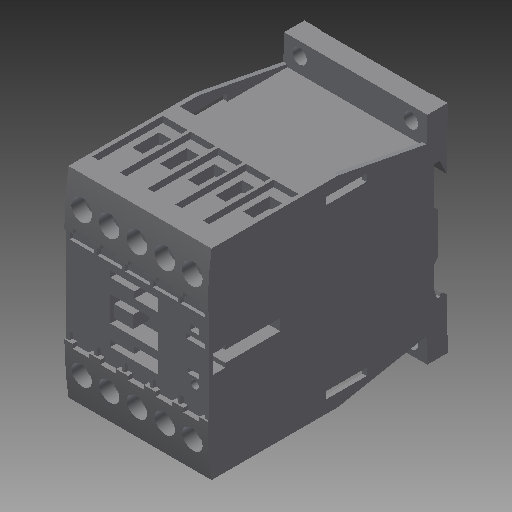
# Autodesk Inventor part: 276845
Saved by Autodesk Inventor 2019.3 (Build 233278000, 278)
## iProperties
Category: PARTsolutions
Company: MOELLER
Created: 2018-10-25
Part Number: 276845
Material: Generic
Catalog Web Link: www.cadenas.de
Description: DC operated-
Vendor: MOELLER
Document SubType Name: Modeling
Designer: psadmin
Manufacturer: MOELLER
Mass: 179.978 g
Surface Area: 287.285 cm^2
Volume: 179.978 cm^3
Density: 1 g/cm^3
Appearance: PSOLRGB-175-175-175
PSOL_IDENT_0: {$CADENAS_DATA\23d-libs\moeller\2\695\733\735\737\740.prj},171 {VTYP=3D},{NB=276845},{LINA=276845},{
PSOL_IDENT_1: NN=DC operated},{DATE=04.10.2018 12:16:44},{GEOMDATE=04.10.2018 08:29:25},{VERSION=v181004082925},{L
PSOL_IDENT_2: INEID=650},{WBVAR=},{WBNUMERIC=}  {NB=276845},{LINA=276845},{KT=DUMMY},{PFOTO=2110pic-214.jpg},{PLID=
PSOL_IDENT_3: 276845},{DATA_SHEET=Data sheet},{MANUTYPEDESC=DILM12-10(24VDC)},{DESCSHORT=Contactor, 3p+1N/O, 5.5kW
PSOL_IDENT_4: /400V/AC3},{DESCLONG=Contactor, Application: Contactors for Motors, Contactors up to 170 A, 3 pole,
PSOL_IDENT_5: Utilization category: AC-1: Non-inductive or slightly inductive loads, resistance furnaces, NAC-3: N
PSOL_IDENT_6: ormal AC induction motors: starting, switch off during running, AC-4: Normal AC induction motors: st
PSOL_IDENT_7: arting, plugging, reversing, inching, Connection technique: Screw terminals, Notes: Also suitable fo
PSOL_IDENT_8: r motors with efficiency class IE3., IE3-ready devices are identified by the logo on their packaging
PSOL_IDENT_9: ., Number of poles: 3 pole, Rated operational current AC-3 380 V 400 V: Ie= 12 A, Rated operational
PSOL_IDENT_10: current AC-1 Conventional free air thermal current, 3 pole, 50 - 60 Hz Open at 40 °C: Ith =Ie= 22 A,
PSOL_IDENT_11: enclosed: Ith= 18 A, Rated operational current AC-1 Conventional free air thermal current, 1 pole o
PSOL_IDENT_12: pen: Ith= 50 A, enclosed: Ith= 45 A, Max. rating for three-phase motors, 50 - 60 Hz AC-3 220 V 230 V
PSOL_IDENT_13: : P= 3.5 kW, 380 V 400 V: P= 5.5 kW, 660 V 690 V: P= 6.5 kW, Max. rating for three-phase motors, 50
PSOL_IDENT_14: - 60 Hz AC-4 220 V 230 V: P= 2 kW, 380 V 400 V: P= 3 kW, 660 V 690 V: P= 4.4 kW, Can be combined wit
PSOL_IDENT_15: h auxiliary contact: DILM32-XHI.., DILA-XHI(V).., Contacts N/O = Normally open: 1 N/O, Instructions:
PSOL_IDENT_16: Contacts to EN 50 012., Integrated varistor suppressor circuit., Voltage AC/DC: DC operation},{EAN=
PSOL_IDENT_17: 4015082768454},{ECLASS_8_1=27-37-10-03},{PACKAGED_WEIGHT=0.296},{DATA_SHEET_=http://datasheet.moelle
PSOL_IDENT_18: r.net/datasheet.php?model=276845&locale=en_GB},{DATA_SHEET_ENG=http://datasheet.moeller.net/datashee
PSOL_IDENT_19: t.php?model=276845&locale=en_GB},{DATA_SHEET_DEU=http://datasheet.moeller.net/datasheet.php?model=27
PSOL_IDENT_20: 6845&locale=de_DE}
NN: DC operated
NB: 276845
NBSYN: $PLID.
LINA: 276845
PFOTO: 2110pic-214.jpg
PLID: 276845
DATA_SHEET: Data sheet
MANUTYPEDESC: DILM12-10(24VDC)
DESCSHORT: Contactor, 3p+1N/O, 5.5kW/400V/AC3
DESCLONG: Contactor, Application: Contactors for Motors, Contactors up to 170 A, 3 pole, Utilization category: AC-1: Non-inductive or slightly inductive loads, resistance furnaces, NAC-3: Normal AC induction motors: starting, switch off during running, AC-4: Normal AC induction motors: starting, plugging, reversing, inching, Connection technique: Screw terminals, Notes: Also suitable for motors with efficiency class IE3., IE3-ready devices are identified by the logo on their packaging., Number of poles: 3 pole, Rated operational current AC-3 380 V 400 V: Ie= 12 A, Rated operational current AC-1 Conventional free air thermal current, 3 pole, 50 - 60 Hz Open at 40 °C: Ith =Ie= 22 A, enclosed: Ith= 18 A, Rated operational current AC-1 Conventional free air thermal current, 1 pole open: Ith= 50 A, enclosed: Ith= 45 A, Max. rating for three-phase motors, 50 - 60 Hz AC-3 220 V 230 V: P= 3.5 kW, 380 V 400 V: P= 5.5 kW, 660 V 690 V: P= 6.5 kW, Max. rating for three-phase motors, 50 - 60 Hz AC-4 220 V 230 V: P= 2 kW, 380 V 400 V: P= 3 kW, 660 V 690 V: P= 4.4 kW, Can be combined with auxiliary contact: DILM32-XHI.., DILA-XHI(V).., Contacts N/O = Normally open: 1 N/O, Instructions: Contacts to EN 50 012., Integrated varistor suppressor circuit., Voltage AC/DC: DC operation
EAN: 4015082768454
ECLASS_8_1: 27-37-10-03
PACKAGED_WEIGHT: 0.296
SUPPLIER: MOELLER
ARTICLENO: 276845
BOMINFO: 276845
CREATOR: CADENAS GmbH
Title: 276845
Author: Cadenas PARTsolutions
Autodesk Inventor part; units mm, degrees
sketch "Sketch_1" plane through (0, 0, 0) normal (1, 0, 0) x (0, 1, 0)
  arc A0 (-15, 72.4777) -> (-31.5, 71.2047) centre (-12.5, -67.5) ccw
  line L0 (-31.5, 71.2047) -> (-31.5, 31.404)
  line L1 (-31.5, 31.404) -> (-26.1094, 3.6715)
  line L2 (-26.1094, 3.6715) -> (-34, 3.396)
  line L3 (-34, 3.396) -> (-34, -3)
  line L4 (-34, -3) -> (-17.9929, -3)
  line L5 (-17.9929, -3) -> (-16.5, -0.8679)
  line L6 (-16.5, -0.8679) -> (-17.5, -0.6)
  line L7 (-17.5, -0.6) -> (-17.5, 0.3)
  line L8 (-17.5, 0.3) -> (-15.0273, 1.2)
  line L9 (-15.0273, 1.2) -> (-7.7, 1.2)
  line L10 (-7.7, 1.2) -> (-6.5, 0)
  line L11 (-6.5, 0) -> (6.5, 0)
  line L12 (6.5, 0) -> (7.7, 1.2)
  line L13 (7.7, 1.2) -> (19.5, 1.2)
  line L14 (19.5, 1.2) -> (19.5, -0.5)
  line L15 (19.5, -0.5) -> (15, -2.5984)
  line L16 (15, -2.5984) -> (15, -3)
  line L17 (15, -3) -> (34, -3)
  line L18 (34, -3) -> (34, 3.396)
  line L19 (34, 3.396) -> (26.1094, 3.6715)
  line L20 (26.1094, 3.6715) -> (31.5, 31.404)
  line L21 (31.5, 31.404) -> (31.5, 71.2047)
  arc A1 (31.5, 71.2047) -> (15, 72.4777) centre (12.5, -67.5) ccw
  line L22 (15, 72.4777) -> (15, 72)
  line L23 (15, 72) -> (-15, 72)
  line L24 (-15, 72) -> (-15, 72.4777)
  line L25 (27.55, 35.25) -> (25.3, 35.25)
  line L26 (25.3, 35.25) -> (25.3, 22.5)
  line L27 (25.3, 22.5) -> (27.55, 22.5)
  line L28 (27.55, 22.5) -> (27.55, 35.25)
  line L29 (-27.55, 35.25) -> (-27.55, 22.5)
  line L30 (-27.55, 22.5) -> (-25.3, 22.5)
  line L31 (-25.3, 22.5) -> (-25.3, 35.25)
  line L32 (-25.3, 35.25) -> (-27.55, 35.25)
  constraints: 66 end point, 4 point on circle, 2 centre point
extrude "Extrusion1" add sketch "Sketch_1" along normal blind 45
sketch "Sketch_77" plane through (0, 0, -3) normal (0, 0, 1) x (1, 0, 0)
  line L0 (0, 29) -> (0, -29)
  line L1 (0, -29) -> (1.3, -29)
  line L2 (1.3, -29) -> (1.3, -32.7)
  line L3 (1.3, -32.7) -> (5, -32.7)
  line L4 (5, -32.7) -> (5, -34)
  line L5 (5, -34) -> (40, -34)
  line L6 (40, -34) -> (40, -32.7)
  line L7 (40, -32.7) -> (43.7, -32.7)
  line L8 (43.7, -32.7) -> (43.7, -29)
  line L9 (43.7, -29) -> (45, -29)
  line L10 (45, -29) -> (45, 29)
  line L11 (45, 29) -> (43.7, 29)
  line L12 (43.7, 29) -> (43.7, 32.7)
  line L13 (43.7, 32.7) -> (40, 32.7)
  line L14 (40, 32.7) -> (40, 34)
  line L15 (40, 34) -> (5, 34)
  line L16 (5, 34) -> (5, 32.7)
  line L17 (5, 32.7) -> (1.3, 32.7)
  line L18 (1.3, 32.7) -> (1.3, 29)
  line L19 (1.3, 29) -> (0, 29)
  constraints: 40 end point
extrude "Extrusion2" cut sketch "Sketch_77" along normal mid plane 0.4
sketch "Sketch_2" plane through (0, 0, -5) normal (0, 0, 1) x (1, 0, 0)
  line L0 (15, -44) -> (30, -44)
  line L1 (30, -44) -> (30, -10)
  line L2 (30, -10) -> (15, -10)
  line L3 (15, -10) -> (15, -44)
  constraints: 8 end point
extrude "Extrusion3" cut sketch "Sketch_2" along normal blind 6.2
sketch "Sketch_3" plane through (0, 0, 0) normal (0, 0, 1) x (1, 0, 0)
  line L0 (14.8, -59.3) -> (30.2, -59.3)
  line L1 (30.2, -59.3) -> (30.2, -25.3)
  line L2 (30.2, -25.3) -> (14.8, -25.3)
  line L3 (14.8, -25.3) -> (14.8, -59.3)
  constraints: 8 end point
extrude "Extrusion4" cut sketch "Sketch_3" along normal mid plane 10
sketch "Sketch_4" plane through (22.5, 0, 0) normal (1, 0, 0) x (0, 0, -1)
  line L0 (-37.5, 25.3) -> (-3.6998, 25.3)
  line L1 (-3.6998, 25.3) -> (-3.396, 34)
  line L2 (-3.396, 34) -> (-37.5, 34)
  line L3 (-37.5, 34) -> (-37.5, 25.3)
  constraints: 8 end point
extrude "Extrusion5" cut sketch "Sketch_4" along normal mid plane 42.4
sketch "Sketch_5" plane through (22.5, 0, 0) normal (1, 0, 0) x (0, 0, -1)
  line L0 (-37.5, -25.3) -> (-37.5, -34)
  line L1 (-37.5, -34) -> (-3.396, -34)
  line L2 (-3.396, -34) -> (-3.6998, -25.3)
  line L3 (-3.6998, -25.3) -> (-37.5, -25.3)
  constraints: 8 end point
extrude "Extrusion6" cut sketch "Sketch_5" along normal mid plane 42.4
sketch "Sketch_6" plane through (0, 0, 0) normal (0, 0, 1) x (1, 0, 0)
  circle A0 centre (22.5, 0) radius 4
  constraints: 1 centre point
extrude "Extrusion7" add sketch "Sketch_6" against normal blind 1
sketch "Sketch_7" plane through (0, 31.5, 0) normal (0, 1, 0) x (1, 0, 0)
  line L0 (1.2, -42.7) -> (1.2, -64.9)
  line L1 (1.2, -64.9) -> (9, -64.9)
  line L2 (9, -64.9) -> (9, -42.7)
  line L3 (9, -42.7) -> (1.2, -42.7)
  constraints: 8 end point
extrude "Extrusion8" cut sketch "Sketch_7" against normal blind 2
sketch "Sketch_8" plane through (0, 31.5, 0) normal (0, 1, 0) x (1, 0, 0)
  line L0 (9.9, -42.7) -> (9.9, -64.9)
  line L1 (9.9, -64.9) -> (17.7, -64.9)
  line L2 (17.7, -64.9) -> (17.7, -42.7)
  line L3 (17.7, -42.7) -> (9.9, -42.7)
  constraints: 8 end point
extrude "Extrusion9" cut sketch "Sketch_8" against normal blind 2
sketch "Sketch_9" plane through (0, 31.5, 0) normal (0, 1, 0) x (1, 0, 0)
  line L0 (18.6, -42.7) -> (18.6, -64.9)
  line L1 (18.6, -64.9) -> (26.4, -64.9)
  line L2 (26.4, -64.9) -> (26.4, -42.7)
  line L3 (26.4, -42.7) -> (18.6, -42.7)
  constraints: 8 end point
extrude "Extrusion10" cut sketch "Sketch_9" against normal blind 2
sketch "Sketch_10" plane through (0, 31.5, 0) normal (0, 1, 0) x (1, 0, 0)
  line L0 (27.3, -42.7) -> (27.3, -64.9)
  line L1 (27.3, -64.9) -> (35.1, -64.9)
  line L2 (35.1, -64.9) -> (35.1, -42.7)
  line L3 (35.1, -42.7) -> (27.3, -42.7)
  constraints: 8 end point
extrude "Extrusion11" cut sketch "Sketch_10" against normal blind 2
sketch "Sketch_11" plane through (0, 31.5, 0) normal (0, 1, 0) x (1, 0, 0)
  line L0 (36, -42.7) -> (36, -64.9)
  line L1 (36, -64.9) -> (43.8, -64.9)
  line L2 (43.8, -64.9) -> (43.8, -42.7)
  line L3 (43.8, -42.7) -> (36, -42.7)
  constraints: 8 end point
extrude "Extrusion12" cut sketch "Sketch_11" against normal blind 2
sketch "Sketch_12" plane through (0, -31.5, 0) normal (0, 1, 0) x (1, 0, 0)
  line L0 (1.2, -42.7) -> (1.2, -64.9)
  line L1 (1.2, -64.9) -> (9, -64.9)
  line L2 (9, -64.9) -> (9, -42.7)
  line L3 (9, -42.7) -> (1.2, -42.7)
  constraints: 8 end point
sketch "Sketch_13" plane through (0, -31.5, 0) normal (0, 1, 0) x (1, 0, 0)
  line L0 (9.9, -42.7) -> (9.9, -64.9)
  line L1 (9.9, -64.9) -> (17.7, -64.9)
  line L2 (17.7, -64.9) -> (17.7, -42.7)
  line L3 (17.7, -42.7) -> (9.9, -42.7)
  constraints: 8 end point
sketch "Sketch_14" plane through (0, -31.5, 0) normal (0, 1, 0) x (1, 0, 0)
  line L0 (18.6, -42.7) -> (18.6, -64.9)
  line L1 (18.6, -64.9) -> (26.4, -64.9)
  line L2 (26.4, -64.9) -> (26.4, -42.7)
  line L3 (26.4, -42.7) -> (18.6, -42.7)
  constraints: 8 end point
sketch "Sketch_15" plane through (0, -31.5, 0) normal (0, 1, 0) x (1, 0, 0)
  line L0 (27.3, -42.7) -> (27.3, -64.9)
  line L1 (27.3, -64.9) -> (35.1, -64.9)
  line L2 (35.1, -64.9) -> (35.1, -42.7)
  line L3 (35.1, -42.7) -> (27.3, -42.7)
  constraints: 8 end point
sketch "Sketch_16" plane through (0, -31.5, 0) normal (0, 1, 0) x (1, 0, 0)
  line L0 (36, -42.7) -> (36, -64.9)
  line L1 (36, -64.9) -> (43.8, -64.9)
  line L2 (43.8, -64.9) -> (43.8, -42.7)
  line L3 (43.8, -42.7) -> (36, -42.7)
  constraints: 8 end point
extrude "Extrusion13" cut sketch "Sketch_12" along normal blind 2
extrude "Extrusion14" cut sketch "Sketch_13" along normal blind 2
extrude "Extrusion15" cut sketch "Sketch_16" along normal blind 2
extrude "Extrusion16" cut sketch "Sketch_15" along normal blind 2
extrude "Extrusion17" cut sketch "Sketch_14" along normal blind 2
sketch "Sketch_17" plane through (0, 31.5, 0) normal (0, 1, 0) x (1, 0, 0)
  line L0 (3.1, -45.8) -> (3.1, -54.2)
  line L1 (3.1, -54.2) -> (7.1, -54.2)
  line L2 (7.1, -54.2) -> (7.1, -45.8)
  line L3 (7.1, -45.8) -> (3.1, -45.8)
  constraints: 8 end point
extrude "Extrusion18" cut sketch "Sketch_17" against normal blind 5.3
sketch "Sketch_18" plane through (0, 31.5, 0) normal (0, 1, 0) x (1, 0, 0)
  line L0 (11.8, -45.8) -> (11.8, -54.2)
  line L1 (11.8, -54.2) -> (15.8, -54.2)
  line L2 (15.8, -54.2) -> (15.8, -45.8)
  line L3 (15.8, -45.8) -> (11.8, -45.8)
  constraints: 8 end point
extrude "Extrusion19" cut sketch "Sketch_18" against normal blind 5.3
sketch "Sketch_19" plane through (0, 31.5, 0) normal (0, 1, 0) x (1, 0, 0)
  line L0 (20.5, -45.8) -> (20.5, -54.2)
  line L1 (20.5, -54.2) -> (24.5, -54.2)
  line L2 (24.5, -54.2) -> (24.5, -45.8)
  line L3 (24.5, -45.8) -> (20.5, -45.8)
  constraints: 8 end point
extrude "Extrusion20" cut sketch "Sketch_19" against normal blind 5.3
sketch "Sketch_20" plane through (0, 31.5, 0) normal (0, 1, 0) x (1, 0, 0)
  line L0 (29.2, -45.8) -> (29.2, -54.2)
  line L1 (29.2, -54.2) -> (33.2, -54.2)
  line L2 (33.2, -54.2) -> (33.2, -45.8)
  line L3 (33.2, -45.8) -> (29.2, -45.8)
  constraints: 8 end point
extrude "Extrusion21" cut sketch "Sketch_20" against normal blind 5.3
sketch "Sketch_21" plane through (0, 31.5, 0) normal (0, 1, 0) x (1, 0, 0)
  line L0 (37.9, -45.8) -> (37.9, -54.2)
  line L1 (37.9, -54.2) -> (41.9, -54.2)
  line L2 (41.9, -54.2) -> (41.9, -45.8)
  line L3 (41.9, -45.8) -> (37.9, -45.8)
  constraints: 8 end point
extrude "Extrusion22" cut sketch "Sketch_21" against normal blind 5.3
sketch "Sketch_22" plane through (0, -31.5, 0) normal (0, 1, 0) x (1, 0, 0)
  line L0 (3.1, -45.8) -> (3.1, -54.2)
  line L1 (3.1, -54.2) -> (7.1, -54.2)
  line L2 (7.1, -54.2) -> (7.1, -45.8)
  line L3 (7.1, -45.8) -> (3.1, -45.8)
  constraints: 8 end point
extrude "Extrusion23" cut sketch "Sketch_22" along normal blind 5.3
sketch "Sketch_23" plane through (0, -31.5, 0) normal (0, 1, 0) x (1, 0, 0)
  line L0 (37.9, -45.8) -> (37.9, -54.2)
  line L1 (37.9, -54.2) -> (41.9, -54.2)
  line L2 (41.9, -54.2) -> (41.9, -45.8)
  line L3 (41.9, -45.8) -> (37.9, -45.8)
  constraints: 8 end point
extrude "Extrusion24" cut sketch "Sketch_23" along normal blind 5.3
sketch "Sketch_24" plane through (0, -31.5, 0) normal (0, 1, 0) x (1, 0, 0)
  line L0 (29.2, -45.8) -> (29.2, -54.2)
  line L1 (29.2, -54.2) -> (33.2, -54.2)
  line L2 (33.2, -54.2) -> (33.2, -45.8)
  line L3 (33.2, -45.8) -> (29.2, -45.8)
  constraints: 8 end point
extrude "Extrusion25" cut sketch "Sketch_24" along normal blind 5.3
sketch "Sketch_25" plane through (0, -31.5, 0) normal (0, 1, 0) x (1, 0, 0)
  line L0 (20.5, -45.8) -> (20.5, -54.2)
  line L1 (20.5, -54.2) -> (24.5, -54.2)
  line L2 (24.5, -54.2) -> (24.5, -45.8)
  line L3 (24.5, -45.8) -> (20.5, -45.8)
  constraints: 8 end point
extrude "Extrusion26" cut sketch "Sketch_25" along normal blind 5.3
sketch "Sketch_26" plane through (0, -31.5, 0) normal (0, 1, 0) x (1, 0, 0)
  line L0 (11.8, -45.8) -> (11.8, -54.2)
  line L1 (11.8, -54.2) -> (15.8, -54.2)
  line L2 (15.8, -54.2) -> (15.8, -45.8)
  line L3 (15.8, -45.8) -> (11.8, -45.8)
  constraints: 8 end point
extrude "Extrusion27" cut sketch "Sketch_26" along normal blind 5.3
sketch "Sketch_27" plane through (0, 0, 66.95) normal (0, 0, 1) x (1, 0, 0)
  circle A0 centre (5.1, 22.5) radius 3.2
  constraints: 1 centre point
extrude "Extrusion28" cut sketch "Sketch_27" along normal blind 10
sketch "Sketch_52" plane through (0, 0, 66.95) normal (0, 0, 1) x (1, 0, 0)
  circle A0 centre (13.8, -22.5) radius 3.2
  constraints: 1 centre point
extrude "Extrusion29" cut sketch "Sketch_52" along normal blind 10
sketch "Sketch_28" plane through (0, 0, 66.95) normal (0, 0, 1) x (1, 0, 0)
  circle A0 centre (13.8, 22.5) radius 3.2
  constraints: 1 centre point
extrude "Extrusion30" cut sketch "Sketch_28" along normal blind 10
sketch "Sketch_46" plane through (0, 0, 66.95) normal (0, 0, 1) x (1, 0, 0)
  circle A0 centre (22.5, 22.5) radius 3.2
  constraints: 1 centre point
extrude "Extrusion31" cut sketch "Sketch_46" along normal blind 10
sketch "Sketch_47" plane through (0, 0, 66.95) normal (0, 0, 1) x (1, 0, 0)
  circle A0 centre (31.2, 22.5) radius 3.2
  constraints: 1 centre point
extrude "Extrusion32" cut sketch "Sketch_47" along normal blind 10
sketch "Sketch_48" plane through (0, 0, 66.95) normal (0, 0, 1) x (1, 0, 0)
  circle A0 centre (39.9, 22.5) radius 3.2
  constraints: 1 centre point
extrude "Extrusion33" cut sketch "Sketch_48" along normal blind 10
sketch "Sketch_49" plane through (0, 0, 66.95) normal (0, 0, 1) x (1, 0, 0)
  circle A0 centre (39.9, -22.5) radius 3.2
  constraints: 1 centre point
extrude "Extrusion34" cut sketch "Sketch_49" along normal blind 10
sketch "Sketch_50" plane through (0, 0, 66.95) normal (0, 0, 1) x (1, 0, 0)
  circle A0 centre (31.2, -22.5) radius 3.2
  constraints: 1 centre point
extrude "Extrusion35" cut sketch "Sketch_50" along normal blind 10
sketch "Sketch_51" plane through (0, 0, 66.95) normal (0, 0, 1) x (1, 0, 0)
  circle A0 centre (22.5, -22.5) radius 3.2
  constraints: 1 centre point
extrude "Extrusion36" cut sketch "Sketch_51" along normal blind 10
sketch "Sketch_53" plane through (0, 0, 66.95) normal (0, 0, 1) x (1, 0, 0)
  circle A0 centre (5.1, -22.5) radius 3.2
  constraints: 1 centre point
extrude "Extrusion37" cut sketch "Sketch_53" along normal blind 10
sketch "Sketch_29" plane through (0, 0, 66.95) normal (0, 0, 1) x (1, 0, 0)
  circle A0 centre (5.1, 22.5) radius 3.8
  line L0 (2.825, 23) -> (2.825, 22)
  line L1 (2.825, 22) -> (4.6, 22)
  line L2 (4.6, 22) -> (4.6, 19.2)
  line L3 (4.6, 19.2) -> (5.6, 19.2)
  line L4 (5.6, 19.2) -> (5.6, 22)
  line L5 (5.6, 22) -> (7.375, 22)
  line L6 (7.375, 22) -> (7.375, 23)
  line L7 (7.375, 23) -> (5.6, 23)
  line L8 (5.6, 23) -> (5.6, 25.8)
  line L9 (5.6, 25.8) -> (4.6, 25.8)
  line L10 (4.6, 25.8) -> (4.6, 23)
  line L11 (4.6, 23) -> (2.825, 23)
  constraints: 24 end point, 1 centre point
extrude "Extrusion38" add sketch "Sketch_29" along normal blind 1.1
sketch "Sketch_31" plane through (0, 0, 71) normal (0, 0, 1) x (1, 0, 0)
  line L0 (1.2, 15) -> (1.2, 12.5)
  line L1 (1.2, 12.5) -> (9, 12.5)
  line L2 (9, 12.5) -> (9, 15)
  line L3 (9, 15) -> (7.6, 15)
  line L4 (7.6, 15) -> (7.6, 16.3)
  line L5 (7.6, 16.3) -> (2.6, 16.3)
  line L6 (2.6, 16.3) -> (2.6, 15)
  line L7 (2.6, 15) -> (1.2, 15)
  constraints: 16 end point
extrude "Extrusion39" cut sketch "Sketch_31" along normal blind 6
sketch "Sketch_33" plane through (0, 0, 71) normal (0, 0, 1) x (1, 0, 0)
  line L0 (1.2, -15) -> (2.6, -15)
  line L1 (2.6, -15) -> (2.6, -16.3)
  line L2 (2.6, -16.3) -> (7.6, -16.3)
  line L3 (7.6, -16.3) -> (7.6, -15)
  line L4 (7.6, -15) -> (9, -15)
  line L5 (9, -15) -> (9, -12.5)
  line L6 (9, -12.5) -> (1.2, -12.5)
  line L7 (1.2, -12.5) -> (1.2, -15)
  constraints: 16 end point
extrude "Extrusion40" cut sketch "Sketch_33" along normal blind 6
sketch "Sketch_35" plane through (0, 0, 72) normal (0, 0, 1) x (1, 0, 0)
  line L0 (14, 4) -> (14, -4)
  line L1 (14, -4) -> (29, -4)
  line L2 (29, -4) -> (29, 4)
  line L3 (29, 4) -> (14, 4)
  line L4 (15.15, 1.95) -> (15.15, -1.95)
  line L5 (15.15, -1.95) -> (21.15, -1.95)
  line L6 (21.15, -1.95) -> (21.15, 1.95)
  line L7 (21.15, 1.95) -> (15.15, 1.95)
  constraints: 16 end point
extrude "Extrusion41" cut sketch "Sketch_35" against normal blind 5
sketch "Sketch_36" plane through (0, 0, 72) normal (0, 0, 1) x (1, 0, 0)
  line L0 (14, 8.5) -> (21.5, 8.5)
  line L1 (21.5, 8.5) -> (21.5, 6.5)
  line L2 (21.5, 6.5) -> (29, 6.5)
  line L3 (29, 6.5) -> (29, 10.4)
  line L4 (29, 10.4) -> (14, 10.4)
  line L5 (14, 10.4) -> (14, 8.5)
  constraints: 12 end point
extrude "Extrusion42" cut sketch "Sketch_36" against normal blind 5
sketch "Sketch_37" plane through (0, 0, 72) normal (0, 0, 1) x (1, 0, 0)
  line L0 (14, -8.5) -> (14, -10.4)
  line L1 (14, -10.4) -> (29, -10.4)
  line L2 (29, -10.4) -> (29, -6.5)
  line L3 (29, -6.5) -> (21.5, -6.5)
  line L4 (21.5, -6.5) -> (21.5, -8.5)
  line L5 (21.5, -8.5) -> (14, -8.5)
  constraints: 12 end point
extrude "Extrusion43" cut sketch "Sketch_37" against normal blind 5
sketch "Sketch_38" plane through (0, 0, 72) normal (0, 0, 1) x (1, 0, 0)
  line L0 (37.9, 5.3) -> (37.9, 3.9)
  line L1 (37.9, 3.9) -> (43.6, 3.9)
  line L2 (43.6, 3.9) -> (43.6, 5.3)
  line L3 (43.6, 5.3) -> (37.9, 5.3)
  constraints: 8 end point
extrude "Extrusion44" cut sketch "Sketch_38" against normal blind 4
sketch "Sketch_78" plane through (0, 0, 72) normal (0, 0, 1) x (1, 0, 0)
  line L0 (39, 8.4) -> (39, 6.7)
  line L1 (39, 6.7) -> (42, 6.7)
  line L2 (42, 6.7) -> (42, 8.4)
  line L3 (42, 8.4) -> (39, 8.4)
  constraints: 8 end point
extrude "Extrusion45" cut sketch "Sketch_78" against normal blind 4
sketch "Sketch_39" plane through (0, 0, 72) normal (0, 0, 1) x (1, 0, 0)
  line L0 (38.3, -3.9) -> (38.3, -5.3)
  line L1 (38.3, -5.3) -> (41.9, -5.3)
  line L2 (41.9, -5.3) -> (41.9, -3.9)
  line L3 (41.9, -3.9) -> (38.3, -3.9)
  constraints: 8 end point
extrude "Extrusion46" cut sketch "Sketch_39" against normal blind 4
sketch "Sketch47" plane through (0, -15, 72) normal (0, 0, 1) x (1, 0, 0)
  point P0 (40.5, 7.7)
hole "Hole1" at (40.5, -7.3, 72) direction (0, 0, -1) diameter 2.58 depth 4
sketch "Sketch_40" plane through (0, 0, 0) normal (1, 0, 0) x (0, 1, 0)
  line L0 (1.8, 58.6) -> (-1.8, 58.6)
  line L1 (-1.8, 58.6) -> (-1.8, 49.6)
  line L2 (-1.8, 49.6) -> (1.8, 49.6)
  line L3 (1.8, 49.6) -> (1.8, 58.6)
  constraints: 8 end point
extrude "Extrusion47" cut sketch "Sketch_40" along normal blind 1
sketch "Sketch_41" plane through (45, 0, 0) normal (1, 0, 0) x (0, 0, -1)
  line L0 (-70.6, 3.1) -> (-70.6, -3.1)
  line L1 (-70.6, -3.1) -> (-66.85, -3.1)
  line L2 (-66.85, -3.1) -> (-66.85, -1.8)
  line L3 (-66.85, -1.8) -> (-49.6, -1.8)
  line L4 (-49.6, -1.8) -> (-49.6, 1.8)
  line L5 (-49.6, 1.8) -> (-66.85, 1.8)
  line L6 (-66.85, 1.8) -> (-66.85, 3.1)
  line L7 (-66.85, 3.1) -> (-70.6, 3.1)
  constraints: 16 end point
extrude "Extrusion48" cut sketch "Sketch_41" against normal blind 4.45
sketch "Sketch_42" plane through (0, 0, 0) normal (1, 0, 0) x (0, 1, 0)
  line L0 (16.5, 48.7) -> (12, 48.7)
  line L1 (12, 48.7) -> (12, 45.7)
  line L2 (12, 45.7) -> (16.5, 45.7)
  line L3 (16.5, 45.7) -> (16.5, 48.7)
  constraints: 8 end point
extrude "Extrusion49" cut sketch "Sketch_42" along normal blind 5
sketch "Sketch_43" plane through (0, 0, 0) normal (1, 0, 0) x (0, 1, 0)
  line L0 (-12, 48.7) -> (-16.5, 48.7)
  line L1 (-16.5, 48.7) -> (-16.5, 45.7)
  line L2 (-16.5, 45.7) -> (-12, 45.7)
  line L3 (-12, 45.7) -> (-12, 48.7)
  constraints: 8 end point
extrude "Extrusion50" cut sketch "Sketch_43" along normal blind 5
sketch "Sketch_44" plane through (0, 0, 0) normal (0, 0, 1) x (1, 0, 0)
  circle A0 centre (5, 30) radius 2.25
  constraints: 1 centre point
extrude "Extrusion51" cut sketch "Sketch_44" along normal mid plane 10
pattern_linear "Rectangular Pattern1" count 2 spacing 35 along (1, 0, 0) count 2 spacing 60 along (0, -1, 0) of "Extrusion51"
sketch "Sketch_32" plane through (0, 0, 71) normal (0, 0, 1) x (1, 0, 0)
  line L0 (9.9, 15) -> (9.9, 12.5)
  line L1 (9.9, 12.5) -> (17.7, 12.5)
  line L2 (17.7, 12.5) -> (17.7, 15)
  line L3 (17.7, 15) -> (16.3, 15)
  line L4 (16.3, 15) -> (16.3, 16.3)
  line L5 (16.3, 16.3) -> (11.3, 16.3)
  line L6 (11.3, 16.3) -> (11.3, 15)
  line L7 (11.3, 15) -> (9.9, 15)
  constraints: 16 end point
extrude "Extrusion52" cut sketch "Sketch_32" along normal blind 6
sketch "Sketch_54" plane through (0, 0, 71) normal (0, 0, 1) x (1, 0, 0)
  line L0 (18.6, 15) -> (18.6, 12.5)
  line L1 (18.6, 12.5) -> (26.4, 12.5)
  line L2 (26.4, 12.5) -> (26.4, 15)
  line L3 (26.4, 15) -> (25, 15)
  line L4 (25, 15) -> (25, 16.3)
  line L5 (25, 16.3) -> (20, 16.3)
  line L6 (20, 16.3) -> (20, 15)
  line L7 (20, 15) -> (18.6, 15)
  constraints: 16 end point
extrude "Extrusion53" cut sketch "Sketch_54" along normal blind 6
sketch "Sketch_55" plane through (0, 0, 71) normal (0, 0, 1) x (1, 0, 0)
  line L0 (27.3, 15) -> (27.3, 12.5)
  line L1 (27.3, 12.5) -> (35.1, 12.5)
  line L2 (35.1, 12.5) -> (35.1, 15)
  line L3 (35.1, 15) -> (33.7, 15)
  line L4 (33.7, 15) -> (33.7, 16.3)
  line L5 (33.7, 16.3) -> (28.7, 16.3)
  line L6 (28.7, 16.3) -> (28.7, 15)
  line L7 (28.7, 15) -> (27.3, 15)
  constraints: 16 end point
extrude "Extrusion54" cut sketch "Sketch_55" along normal blind 6
sketch "Sketch_56" plane through (0, 0, 71) normal (0, 0, 1) x (1, 0, 0)
  line L0 (36, 15) -> (36, 12.5)
  line L1 (36, 12.5) -> (43.8, 12.5)
  line L2 (43.8, 12.5) -> (43.8, 15)
  line L3 (43.8, 15) -> (42.4, 15)
  line L4 (42.4, 15) -> (42.4, 16.3)
  line L5 (42.4, 16.3) -> (37.4, 16.3)
  line L6 (37.4, 16.3) -> (37.4, 15)
  line L7 (37.4, 15) -> (36, 15)
  constraints: 16 end point
extrude "Extrusion55" cut sketch "Sketch_56" along normal blind 6
sketch "Sketch_34" plane through (0, 0, 71) normal (0, 0, 1) x (1, 0, 0)
  line L0 (9.9, -15) -> (11.3, -15)
  line L1 (11.3, -15) -> (11.3, -16.3)
  line L2 (11.3, -16.3) -> (16.3, -16.3)
  line L3 (16.3, -16.3) -> (16.3, -15)
  line L4 (16.3, -15) -> (17.7, -15)
  line L5 (17.7, -15) -> (17.7, -12.5)
  line L6 (17.7, -12.5) -> (9.9, -12.5)
  line L7 (9.9, -12.5) -> (9.9, -15)
  constraints: 16 end point
extrude "Extrusion56" cut sketch "Sketch_34" along normal blind 6
sketch "Sketch_57" plane through (0, 0, 71) normal (0, 0, 1) x (1, 0, 0)
  line L0 (18.6, -15) -> (20, -15)
  line L1 (20, -15) -> (20, -16.3)
  line L2 (20, -16.3) -> (25, -16.3)
  line L3 (25, -16.3) -> (25, -15)
  line L4 (25, -15) -> (26.4, -15)
  line L5 (26.4, -15) -> (26.4, -12.5)
  line L6 (26.4, -12.5) -> (18.6, -12.5)
  line L7 (18.6, -12.5) -> (18.6, -15)
  constraints: 16 end point
extrude "Extrusion57" cut sketch "Sketch_57" along normal blind 6
sketch "Sketch_58" plane through (0, 0, 71) normal (0, 0, 1) x (1, 0, 0)
  line L0 (27.3, -15) -> (28.7, -15)
  line L1 (28.7, -15) -> (28.7, -16.3)
  line L2 (28.7, -16.3) -> (33.7, -16.3)
  line L3 (33.7, -16.3) -> (33.7, -15)
  line L4 (33.7, -15) -> (35.1, -15)
  line L5 (35.1, -15) -> (35.1, -12.5)
  line L6 (35.1, -12.5) -> (27.3, -12.5)
  line L7 (27.3, -12.5) -> (27.3, -15)
  constraints: 16 end point
extrude "Extrusion58" cut sketch "Sketch_58" along normal blind 6
sketch "Sketch_59" plane through (0, 0, 71) normal (0, 0, 1) x (1, 0, 0)
  line L0 (36, -15) -> (37.4, -15)
  line L1 (37.4, -15) -> (37.4, -16.3)
  line L2 (37.4, -16.3) -> (42.4, -16.3)
  line L3 (42.4, -16.3) -> (42.4, -15)
  line L4 (42.4, -15) -> (43.8, -15)
  line L5 (43.8, -15) -> (43.8, -12.5)
  line L6 (43.8, -12.5) -> (36, -12.5)
  line L7 (36, -12.5) -> (36, -15)
  constraints: 16 end point
extrude "Extrusion59" cut sketch "Sketch_59" along normal blind 6
sketch "Sketch_60" plane through (0, 0, 2.9) normal (0, 0, 1) x (1, 0, 0)
  line L0 (10, -34) -> (13, -34)
  line L1 (13, -34) -> (13, -25.3)
  line L2 (13, -25.3) -> (10, -25.3)
  line L3 (10, -25.3) -> (10, -34)
  constraints: 8 end point
extrude "Extrusion60" cut sketch "Sketch_60" along normal blind 2
sketch "Sketch_61" plane through (0, 0, 2.9) normal (0, 0, 1) x (1, 0, 0)
  line L0 (32, -34) -> (35, -34)
  line L1 (35, -34) -> (35, -25.3)
  line L2 (35, -25.3) -> (32, -25.3)
  line L3 (32, -25.3) -> (32, -34)
  constraints: 8 end point
extrude "Extrusion61" cut sketch "Sketch_61" along normal blind 2
sketch "Sketch_30" plane through (0, 0, 66.95) normal (0, 0, 1) x (1, 0, 0)
  circle A0 centre (13.8, 22.5) radius 3.8
  line L0 (11.525, 23) -> (11.525, 22)
  line L1 (11.525, 22) -> (13.3, 22)
  line L2 (13.3, 22) -> (13.3, 19.2)
  line L3 (13.3, 19.2) -> (14.3, 19.2)
  line L4 (14.3, 19.2) -> (14.3, 22)
  line L5 (14.3, 22) -> (16.075, 22)
  line L6 (16.075, 22) -> (16.075, 23)
  line L7 (16.075, 23) -> (14.3, 23)
  line L8 (14.3, 23) -> (14.3, 25.8)
  line L9 (14.3, 25.8) -> (13.3, 25.8)
  line L10 (13.3, 25.8) -> (13.3, 23)
  line L11 (13.3, 23) -> (11.525, 23)
  constraints: 24 end point, 1 centre point
extrude "Extrusion62" add sketch "Sketch_30" along normal blind 1.1
sketch "Sketch_62" plane through (0, 0, 66.95) normal (0, 0, 1) x (1, 0, 0)
  circle A0 centre (22.5, 22.5) radius 3.8
  line L0 (20.225, 23) -> (20.225, 22)
  line L1 (20.225, 22) -> (22, 22)
  line L2 (22, 22) -> (22, 19.2)
  line L3 (22, 19.2) -> (23, 19.2)
  line L4 (23, 19.2) -> (23, 22)
  line L5 (23, 22) -> (24.775, 22)
  line L6 (24.775, 22) -> (24.775, 23)
  line L7 (24.775, 23) -> (23, 23)
  line L8 (23, 23) -> (23, 25.8)
  line L9 (23, 25.8) -> (22, 25.8)
  line L10 (22, 25.8) -> (22, 23)
  line L11 (22, 23) -> (20.225, 23)
  constraints: 24 end point, 1 centre point
extrude "Extrusion63" add sketch "Sketch_62" along normal blind 1.1
sketch "Sketch_63" plane through (0, 0, 66.95) normal (0, 0, 1) x (1, 0, 0)
  circle A0 centre (31.2, 22.5) radius 3.8
  line L0 (28.925, 23) -> (28.925, 22)
  line L1 (28.925, 22) -> (30.7, 22)
  line L2 (30.7, 22) -> (30.7, 19.2)
  line L3 (30.7, 19.2) -> (31.7, 19.2)
  line L4 (31.7, 19.2) -> (31.7, 22)
  line L5 (31.7, 22) -> (33.475, 22)
  line L6 (33.475, 22) -> (33.475, 23)
  line L7 (33.475, 23) -> (31.7, 23)
  line L8 (31.7, 23) -> (31.7, 25.8)
  line L9 (31.7, 25.8) -> (30.7, 25.8)
  line L10 (30.7, 25.8) -> (30.7, 23)
  line L11 (30.7, 23) -> (28.925, 23)
  constraints: 24 end point, 1 centre point
extrude "Extrusion64" add sketch "Sketch_63" along normal blind 1.1
sketch "Sketch_64" plane through (0, 0, 66.95) normal (0, 0, 1) x (1, 0, 0)
  circle A0 centre (39.9, 22.5) radius 3.8
  line L0 (37.625, 23) -> (37.625, 22)
  line L1 (37.625, 22) -> (39.4, 22)
  line L2 (39.4, 22) -> (39.4, 19.2)
  line L3 (39.4, 19.2) -> (40.4, 19.2)
  line L4 (40.4, 19.2) -> (40.4, 22)
  line L5 (40.4, 22) -> (42.175, 22)
  line L6 (42.175, 22) -> (42.175, 23)
  line L7 (42.175, 23) -> (40.4, 23)
  line L8 (40.4, 23) -> (40.4, 25.8)
  line L9 (40.4, 25.8) -> (39.4, 25.8)
  line L10 (39.4, 25.8) -> (39.4, 23)
  line L11 (39.4, 23) -> (37.625, 23)
  constraints: 24 end point, 1 centre point
extrude "Extrusion65" add sketch "Sketch_64" along normal blind 1.1
sketch "Sketch_65" plane through (0, 0, 66.95) normal (0, 0, 1) x (1, 0, 0)
  circle A0 centre (39.9, -22.5) radius 3.8
  line L0 (37.625, -22) -> (37.625, -23)
  line L1 (37.625, -23) -> (39.4, -23)
  line L2 (39.4, -23) -> (39.4, -25.8)
  line L3 (39.4, -25.8) -> (40.4, -25.8)
  line L4 (40.4, -25.8) -> (40.4, -23)
  line L5 (40.4, -23) -> (42.175, -23)
  line L6 (42.175, -23) -> (42.175, -22)
  line L7 (42.175, -22) -> (40.4, -22)
  line L8 (40.4, -22) -> (40.4, -19.2)
  line L9 (40.4, -19.2) -> (39.4, -19.2)
  line L10 (39.4, -19.2) -> (39.4, -22)
  line L11 (39.4, -22) -> (37.625, -22)
  constraints: 24 end point, 1 centre point
extrude "Extrusion66" add sketch "Sketch_65" along normal blind 1.1
sketch "Sketch_66" plane through (0, 0, 66.95) normal (0, 0, 1) x (1, 0, 0)
  circle A0 centre (31.2, -22.5) radius 3.8
  line L0 (28.925, -22) -> (28.925, -23)
  line L1 (28.925, -23) -> (30.7, -23)
  line L2 (30.7, -23) -> (30.7, -25.8)
  line L3 (30.7, -25.8) -> (31.7, -25.8)
  line L4 (31.7, -25.8) -> (31.7, -23)
  line L5 (31.7, -23) -> (33.475, -23)
  line L6 (33.475, -23) -> (33.475, -22)
  line L7 (33.475, -22) -> (31.7, -22)
  line L8 (31.7, -22) -> (31.7, -19.2)
  line L9 (31.7, -19.2) -> (30.7, -19.2)
  line L10 (30.7, -19.2) -> (30.7, -22)
  line L11 (30.7, -22) -> (28.925, -22)
  constraints: 24 end point, 1 centre point
extrude "Extrusion67" add sketch "Sketch_66" along normal blind 1.1
sketch "Sketch_67" plane through (0, 0, 66.95) normal (0, 0, 1) x (1, 0, 0)
  circle A0 centre (22.5, -22.5) radius 3.8
  line L0 (20.225, -22) -> (20.225, -23)
  line L1 (20.225, -23) -> (22, -23)
  line L2 (22, -23) -> (22, -25.8)
  line L3 (22, -25.8) -> (23, -25.8)
  line L4 (23, -25.8) -> (23, -23)
  line L5 (23, -23) -> (24.775, -23)
  line L6 (24.775, -23) -> (24.775, -22)
  line L7 (24.775, -22) -> (23, -22)
  line L8 (23, -22) -> (23, -19.2)
  line L9 (23, -19.2) -> (22, -19.2)
  line L10 (22, -19.2) -> (22, -22)
  line L11 (22, -22) -> (20.225, -22)
  constraints: 24 end point, 1 centre point
extrude "Extrusion68" add sketch "Sketch_67" along normal blind 1.1
sketch "Sketch_68" plane through (0, 0, 66.95) normal (0, 0, 1) x (1, 0, 0)
  circle A0 centre (13.8, -22.5) radius 3.8
  line L0 (11.525, -22) -> (11.525, -23)
  line L1 (11.525, -23) -> (13.3, -23)
  line L2 (13.3, -23) -> (13.3, -25.8)
  line L3 (13.3, -25.8) -> (14.3, -25.8)
  line L4 (14.3, -25.8) -> (14.3, -23)
  line L5 (14.3, -23) -> (16.075, -23)
  line L6 (16.075, -23) -> (16.075, -22)
  line L7 (16.075, -22) -> (14.3, -22)
  line L8 (14.3, -22) -> (14.3, -19.2)
  line L9 (14.3, -19.2) -> (13.3, -19.2)
  line L10 (13.3, -19.2) -> (13.3, -22)
  line L11 (13.3, -22) -> (11.525, -22)
  constraints: 24 end point, 1 centre point
extrude "Extrusion69" add sketch "Sketch_68" along normal blind 1.1
sketch "Sketch_69" plane through (0, 0, 66.95) normal (0, 0, 1) x (1, 0, 0)
  circle A0 centre (5.1, -22.5) radius 3.8
  line L0 (2.825, -22) -> (2.825, -23)
  line L1 (2.825, -23) -> (4.6, -23)
  line L2 (4.6, -23) -> (4.6, -25.8)
  line L3 (4.6, -25.8) -> (5.6, -25.8)
  line L4 (5.6, -25.8) -> (5.6, -23)
  line L5 (5.6, -23) -> (7.375, -23)
  line L6 (7.375, -23) -> (7.375, -22)
  line L7 (7.375, -22) -> (5.6, -22)
  line L8 (5.6, -22) -> (5.6, -19.2)
  line L9 (5.6, -19.2) -> (4.6, -19.2)
  line L10 (4.6, -19.2) -> (4.6, -22)
  line L11 (4.6, -22) -> (2.825, -22)
  constraints: 24 end point, 1 centre point
extrude "Extrusion70" add sketch "Sketch_69" along normal blind 1.1
ref_plane "DIL_M7_15_XY" through (0, 0, 0) normal (0, 0, 1) x (1, 0, 0)
ref_plane "DIL_M7_15_YZ" through (0, 0, 0) normal (1, 0, 0) x (0, 1, 0)
ref_plane "DIL_M7_15_ZX" through (0, 0, 0) normal (0, 1, 0) x (0, 0, 1)
ref_plane "DIL_M7_15_2_XY" through (45, 0, 0) normal (0, 0, 1) x (1, 0, 0)
ref_plane "DIL_M7_15_2_YZ" through (45, 0, 0) normal (1, 0, 0) x (0, 1, 0)
ref_plane "DIL_M7_15_2_ZX" through (45, 0, 0) normal (0, 1, 0) x (0, 0, 1)
ref_plane "XHI_XY" through (18.15, 0, 72) normal (0, 0, -1) x (1, 0, 0)
ref_plane "XHI_YZ" through (18.15, 0, 72) normal (1, 0, 0) x (0, -1, 0)
ref_plane "XHI_ZX" through (18.15, 0, 72) normal (0, -1, 0) x (0, 0, -1)
ref_plane "XHI_S_XY" through (0, 14.25, 47.2) normal (-1, 0, 0) x (0, 0, -1)
ref_plane "XHI_S_YZ" through (0, 14.25, 47.2) normal (0, 0, -1) x (0, -1, 0)
ref_plane "XHI_S_ZX" through (0, 14.25, 47.2) normal (0, -1, 0) x (-1, 0, 0)
ref_plane "XM12_XY" through (22.5, 34, -2.8) normal (0, 0, 1) x (1, 0, 0)
ref_plane "XM12_YZ" through (22.5, 34, -2.8) normal (1, 0, 0) x (0, 1, 0)
ref_plane "XM12_ZX" through (22.5, 34, -2.8) normal (0, 1, 0) x (0, 0, 1)
ref_plane "XMCE_XY" through (22.5, 0, -1) normal (0, 0, 1) x (1, 0, 0)
ref_plane "XMCE_YZ" through (22.5, 0, -1) normal (1, 0, 0) x (0, 1, 0)
ref_plane "XMCE_ZX" through (22.5, 0, -1) normal (0, 1, 0) x (0, 0, 1)
ref_plane "XMV___XY" through (45, 0, 68.3) normal (1, 0, 0) x (0, 0, -1)
ref_plane "XMV___YZ" through (45, 0, 68.3) normal (0, 0, -1) x (0, 1, 0)
ref_plane "XMV___ZX" through (45, 0, 68.3) normal (0, 1, 0) x (1, 0, 0)
ref_plane "XSP_XY" through (45, 0, 72) normal (1, 0, 0) x (0, 0, -1)
ref_plane "XSP_YZ" through (45, 0, 72) normal (0, 0, -1) x (0, 1, 0)
ref_plane "XSP_ZX" through (45, 0, 72) normal (0, 1, 0) x (1, 0, 0)
body "Solid1"
